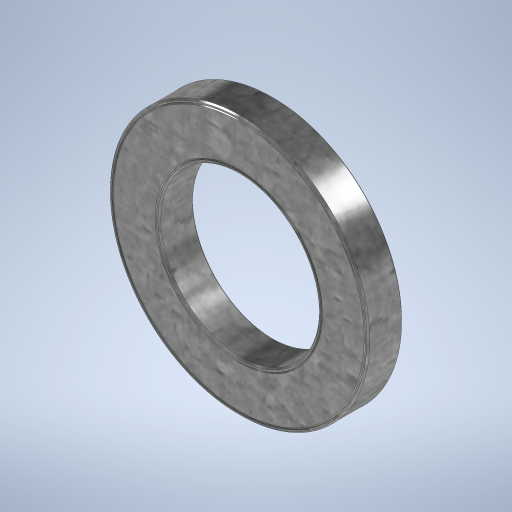
# Autodesk Inventor part: 6203베어링
Saved by Autodesk Inventor 2023 (Build 270158000, 158)
## iProperties
Created: 2022-06-08
Part Number: 6203베어링
Material: 일반
Document SubType Name: Modeling
Designer: fly01
Density: 1 g/cm^3
Appearance: 기본값
Author: fly01
Autodesk Inventor part; units mm, degrees
ref_plane "YZ Plane" through (0, 0, 0) normal (1, 0, 0) x (0, 1, 0)
ref_plane "XZ Plane" through (0, 0, 0) normal (0, 1, 0) x (-1, 0, 0)
ref_plane "XY Plane" through (0, 0, 0) normal (0, 0, 1) x (1, 0, 0)
sketch "스케치1" plane through (0, 0, 0) normal (0, 0, 1) x (1, 0, 0)
  circle A0 centre (0, 0) radius 27.5
  circle A1 centre (0, 0) radius 45
  dimension "d0" = 55
  dimension "d1" = 90
  constraints: 2 centre point, 2 coincident
  measures "d0" diameter of A0
  measures "d1" diameter of A1
extrude "돌출1" add sketch "스케치1" along normal mid plane 12
chamfer "모따기1" distance 0.5 angle 45 4 edges at (-45, 0, 6) (-45, 0, -6) (-27.5, 0, 6) (-27.5, 0, -6)
sketch "스케치2" plane through (0, 0, 0) normal (0, 1, 0) x (-1, 0, 0)
  line L0 (-44.5, 6) -> (44.5, 6) projected
  line L1 (44, 6) -> (44, 5.7414)
  line L2 (43.8293, 5.6707) -> (43.5, 6)
  line L3 (45, 0) -> (27.5, 0)
  line L4 (27.5, 5.5) -> (27.5, -5.5) projected
  arc A0 (43.8293, 5.6707) -> (44, 5.7414) centre (43.9, 5.7414) ccw
  line L5 (36.25, 0) -> (36.25, 1.7292)
  line L6 (28.5, 6) -> (28.5, 5.7414)
  line L7 (28.6707, 5.6707) -> (29, 6)
  arc A1 (28.5, 5.7414) -> (28.6707, 5.6707) centre (28.6, 5.7414) ccw
  line L8 (44, -6) -> (44, -5.7414)
  line L9 (43.8293, -5.6707) -> (43.5, -6)
  arc A2 (44, -5.7414) -> (43.8293, -5.6707) centre (43.9, -5.7414) ccw
  line L10 (28.5, -6) -> (28.5, -5.7414)
  line L11 (28.6707, -5.6707) -> (29, -6)
  arc A3 (28.6707, -5.6707) -> (28.5, -5.7414) centre (28.6, -5.7414) ccw
  line L12 (0, 0) -> (0, -13.1586)
  line L13 (44.5, -6) -> (-44.5, -6) projected
  line L14 (45, -5.5) -> (45, 5.5) projected
  point P0 (44, 5.5)
  point P1 (28, 6)
  point P2 (28.5, 5.5)
  point P3 (44, -5.5)
  point P4 (28, -6)
  point P5 (28.5, -5.5)
  dimension "d7" = 0.5
  dimension "d8" = 0.5
  dimension "d9" = 0.5
  dimension "d10" = 0.1
  constraints: 22 end point, 21 symmetric about line, 10 point on line, 8 point on circle, 4 centre point, 3 midpoint, 3 vertical, 2 tangent, 3 other
  measures "d7" distance of L0.end L1.start
  measures "d8" distance of L1.start point (44, 5.5)
  measures "d9" distance of L1.start L2.end
  measures "d10" radius of A0
revolve "회전1" cut sketch "스케치2" angle 360 about axis through (0, 0, 0) along (0, 0, -1)
